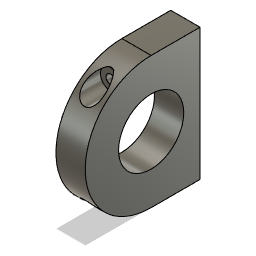
Pedal Mounting Ears v1 (Autodesk Fusion 360 design; units mm, degrees)
Autodesk Fusion 360 part; units mm, degrees
sketch "Sketch1" plane through (0, 0, 0) normal (1, 0, 0) x (0, 0, -1)
  line L0 (-16.6875, 45) -> (0, 45)
  line L1 (0, 45) -> (0, 0)
  line L2 (0, 0) -> (-16.6875, 0)
  arc A0 (-16.6875, 45) -> (-16.6875, 0) centre (-16.6875, 22.5) ccw
  circle A1 centre (-16.6875, 22.5) radius 11.125
  line L3 (0, 22.5) -> (-29, 22.5) construction
  circle A2 centre (-16.6875, 22.5) radius 9.125
  dimension "d1" = 22.25
  dimension "d2" = 45
  dimension "d3" = 16.6875
  dimension "d4" = -2
  constraint horizontal L0
  constraint coincident L1.end L2.start
  constraint perpendicular L0 L1
  constraint perpendicular L1 L2
  constraint tangent L2 A0
  constraint tangent L0 A0
  constraint midpoint L1 L3.start
  constraint perpendicular L1 L3
  constraint coincident A0.centre L3
  constraint coincident A0.centre A1.centre
  measures "d1" diameter of A1
  measures "d2" distance of L0 L2
  measures "d3" distance of L1 A0.centre
extrude "Extrude2" add sketch "Sketch1" along normal blind 10 contours L0 L1 L2 A0
sketch "Sketch2" plane through (0, 0, 0) normal (0, 0, -1) x (-1, 0, 0)
  line L0 (0, 45) -> (-10, 45)
  line L1 (-10, 0) -> (0, 0)
  circle A0 centre (-5, 5.2) radius 3.5
  line L2 (-5, 0) -> (-5, 4) construction
  circle A1 centre (-5, 5.2) radius 1.6
  line L3 (0, 0) -> (0, 45)
  line L4 (-10, 45) -> (-10, 0)
  dimension "d13" = 7
  dimension "d14" = 5.2
  dimension "d17" = 3.2
  constraint midpoint L1 L2.start
  constraint perpendicular L1 L2
  constraint coincident A0.centre L2
  constraint concentric A0 A1
  measures "d13" diameter of A0
  measures "d14" distance of L1 A0.centre
  measures "d17" diameter of A1
extrude "Extrude4" cut sketch "Sketch2" against normal blind 40 contours A0 | A1
extrude "Extrude5" add sketch "Sketch2" against normal blind 25.5 contours A0
ref_plane "WorkPlane1" through (5, 22.5, 8.3438) normal (0, -1, 0) x (0, 0, -1)
mirror "Mirror1" about plane through (5, 22.5, 8.3438) normal (0, -1, 0) of "Extrude4", "Extrude5"
equation "d3 = d1 * 0.75"
equation "d14 = d13 / 2 + 1.7 mm"
